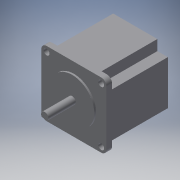
# Autodesk Inventor part: Big Chungus Motor
Saved by Autodesk Inventor 2019 (Build 230136000, 136)
## iProperties
Created: 2022-04-03
Part Number: Big Chungus Motor
Material: Generic
Document SubType Name: Modeling
Designer: Ian
Density: 1 g/cm^3
Appearance: Default
Author: Ian
Autodesk Inventor part; units mm, degrees
ref_plane "YZ Plane" through (0, 0, 0) normal (1, 0, 0) x (0, 1, 0)
ref_plane "XZ Plane" through (0, 0, 0) normal (0, 1, 0) x (-1, 0, 0)
ref_plane "XY Plane" through (0, 0, 0) normal (0, 0, 1) x (1, 0, 0)
sketch "Sketch1" plane through (0, 0, 0) normal (0, 0, 1) x (1, 0, 0)
  line L0 (0, 0) -> (56, 0) construction
  line L1 (56, 0) -> (56, 56) construction
  line L2 (56, 56) -> (0, 56) construction
  line L3 (0, 56) -> (0, 0) construction
  line L4 (0, 47) -> (9, 47)
  line L5 (9, 47) -> (9, 56)
  line L6 (9, 56) -> (47, 56)
  line L7 (47, 56) -> (47, 47)
  line L8 (47, 47) -> (56, 47)
  line L9 (56, 47) -> (56, 9)
  line L10 (56, 9) -> (47, 9)
  line L11 (47, 9) -> (47, 0)
  line L12 (47, 0) -> (9, 0)
  line L13 (9, 0) -> (9, 9)
  line L14 (9, 9) -> (0, 9)
  line L15 (0, 9) -> (0, 47)
  dimension "d0" = 56
  dimension "d1" = 38
  constraints: 32 end point, 16 point on line, 9 perpendicular, 2 horizontal, 2 parallel
  measures "d0" distance of L1.end L2.end
  measures "d1" distance of L5.end L6.end
extrude "Extrusion1" add sketch "Sketch1" along normal blind 48
sketch "Sketch2" plane through (0, 0, 48) normal (0, 0, 1) x (1, 0, 0)
  line L0 (9, 47) -> (0, 47) projected
  line L1 (0, 47) -> (0, 9) projected
  line L2 (0, 9) -> (9, 9) projected
  line L3 (9, 9) -> (9, 0) projected
  line L4 (9, 0) -> (47, 0) projected
  line L5 (47, 0) -> (47, 9) projected
  line L6 (47, 9) -> (56, 9) projected
  line L7 (56, 9) -> (56, 47) projected
  line L8 (56, 47) -> (47, 47) projected
  line L9 (47, 47) -> (47, 56) projected
  line L10 (47, 56) -> (9, 56) projected
  line L11 (9, 56) -> (9, 47) projected
  line L12 (9, 47) -> (0, 47)
  line L13 (0, 47) -> (0, 56)
  line L14 (0, 56) -> (9, 56)
  line L15 (9, 56) -> (9, 47)
  line L16 (47, 47) -> (56, 47) projected
  line L17 (47, 47) -> (56, 47)
  line L18 (56, 47) -> (56, 56)
  line L19 (56, 56) -> (47, 56)
  line L20 (47, 56) -> (47, 47)
  line L21 (47, 9) -> (47, 0) projected
  line L22 (47, 9) -> (56, 9)
  line L23 (56, 9) -> (56, 0)
  line L24 (56, 0) -> (47, 0)
  line L25 (47, 0) -> (47, 9)
  line L26 (47, 0) -> (9, 0) projected
  line L27 (9, 9) -> (0, 9) projected
  line L28 (9, 0) -> (0, 0)
  line L29 (0, 0) -> (0, 9)
  line L30 (0, 9) -> (9, 9)
  line L31 (9, 9) -> (9, 0)
  line L32 (47, 9) -> (56, 9) projected
  line L33 (47, 0) -> (47, 9) projected
  line L34 (47, 47) -> (47, 56) projected
  circle A0 centre (4.5, 51.5) radius 2.5
  circle A1 centre (51.5, 51.5) radius 2.5
  circle A2 centre (51.5, 4.5) radius 2.5
  circle A3 centre (4.5, 4.5) radius 2.5
  line L35 (4.5, 51.5) -> (51.5, 51.5) construction
  line L36 (51.5, 51.5) -> (51.5, 4.5) construction
  line L37 (51.5, 4.5) -> (4.5, 4.5) construction
  line L38 (4.5, 4.5) -> (4.5, 51.5) construction
  line L39 (0, 56) -> (56, 0) construction
  line L40 (47, 47) -> (56, 56) construction
  line L41 (28, 51.5) -> (28, 28) construction
  line L42 (28, 28) -> (4.5, 28) construction
  arc A4 (4.5, 56) -> (0, 51.5) centre (4.5, 51.5) ccw
  arc A5 (56, 51.5) -> (51.5, 56) centre (51.5, 51.5) ccw
  arc A6 (0, 4.5) -> (4.5, 0) centre (4.5, 4.5) ccw
  arc A7 (51.5, 0) -> (56, 4.5) centre (51.5, 4.5) ccw
  dimension "d4" = 5
  dimension "d5" = 47
  constraints: 48 end point, 11 midpoint, 10 parallel, 8 centre point, 8 point on circle, 8 tangent, 7 equal length, 7 perpendicular, 5 horizontal, 3 coincident, 3 equal radius, 2 point on line
  measures "d4" diameter of A0
  measures "d5" distance of L35.start L35.end
extrude "Extrusion2" add sketch "Sketch2" along normal blind 4.8 contours L11 L10 L9 L8 L7 L6 L5 L4 L3 L2 L1 L0 | L0 L13 A4 L14 L11 | L2 L3 L28 A6 L29 | L19 A5 L18 L8 L9 | L5 L6 L23 A7 L24
sketch "Sketch3" plane through (0, 0, 52.8) normal (0, 0, 1) x (1, 0, 0)
  circle A0 centre (28, 28) radius 19
  circle A1 centre (4.5, 4.5) radius 2.5 construction
  circle A2 centre (51.5, 51.5) radius 2.5 construction
  line L0 (4.5, 4.5) -> (51.5, 51.5) construction
  point P0 (0, 0)
  dimension "d8" = 38
  constraints: 2 end point, 1 centre point, 1 coincident, 1 midpoint
  measures "d8" diameter of A0
extrude "Extrusion3" add sketch "Sketch3" along normal blind 1.5
sketch "Sketch4" plane through (28, 28, 54.3) normal (0, 0, 1) x (1, 0, 0)
  circle A0 centre (0, 0) radius 3.15
  point P0 (-28, -28)
  dimension "d11" = 6.3
  constraints: 1 centre point
  measures "d11" diameter of A0
extrude "Extrusion4" add sketch "Sketch4" along normal blind 6.6
sketch "Sketch5" plane through (28, 28, 60.9) normal (0, 0, 1) x (1, 0, 0)
  circle A0 centre (0, 0) radius 3.15 projected
  line L0 (-2.4739, -1.95) -> (2.4739, -1.95)
  circle A1 centre (0, 0) radius 3.15 projected
  point P0 (-28, -28)
  dimension "d14" = 5.1
  constraints: 2 end point, 1 horizontal, 1 point on circle, 2 other
extrude "Extrusion5" add sketch "Sketch5" along normal blind 17 contours A0 L0 picked at (0.6783, 0.1866)
body "Solid1"
